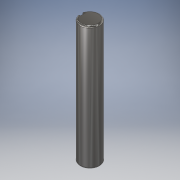
# Autodesk Inventor part: keyed shaft 80mm
Saved by Autodesk Inventor 2019 (Build 230136000, 136)
## iProperties
Created: 2018-08-04
Part Number: keyed shaft 80mm
Material: Steel, High Strength, Low Alloy
Document SubType Name: Modeling
Designer: torba
Density: 7.85 g/cm^3
Appearance: Steel - Polished
Author: torba
Autodesk Inventor part; units mm, degrees
ref_plane "YZ Plane" through (0, 0, 0) normal (1, 0, 0) x (0, 1, 0)
ref_plane "XZ Plane" through (0, 0, 0) normal (0, 1, 0) x (-1, 0, 0)
ref_plane "XY Plane" through (0, 0, 0) normal (0, 0, 1) x (1, 0, 0)
sketch "Sketch1" plane through (0, 0, 0) normal (0, 1, 0) x (-1, 0, 0)
  arc A0 (6.1484, 1.5875) -> (6.1484, -1.5875) centre (0, 0) ccw
  line L0 (4.572, 1.5875) -> (9.2155, 1.5875)
  line L1 (9.2155, 1.5875) -> (9.2155, -1.5875)
  line L2 (9.2155, -1.5875) -> (4.572, -1.5875)
  line L3 (4.572, -1.5875) -> (4.572, 1.5875)
  line L4 (4.572, 1.5875) -> (9.2155, -1.5875) construction
  line L5 (9.2155, 1.5875) -> (4.572, -1.5875) construction
  dimension "d0" = 12.7
  dimension "d1" = 3.175
  dimension "d2" = 55.638
  dimension "d4" = 1.5875
  dimension "d5" = 10.922
  constraints: 12 end point, 2 parallel, 2 point on circle, 2 point on line, 1 centre point, 1 coincident, 1 horizontal, 1 perpendicular
  measures "d0" diameter of A0
  measures "d1" distance of L0.end L1.end
  measures "d2" angle of L5 L1
  measures "d4" distance from line of point (0, 0) L0
extrude "Extrusion1" add sketch "Sketch1" along normal blind 80 contours L0 L3 L2 A0
fillet "Fillet1" radius 1 2 edges at (6.35, 80, 0) (6.35, 0, 0)
body "Solid1"
